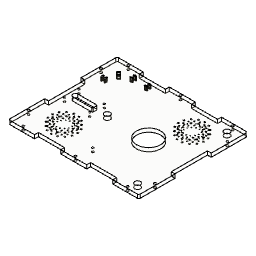
carter_dessous_KOSMOS3-0 (Autodesk Fusion 360 design; units mm, degrees)
Autodesk Fusion 360 part; units mm, degrees
sketch "Esquisse1" plane through (0, 0, 0) normal (0, 0, 1) x (1, 0, 0)
  circle A0 centre (-16.5, 75) radius 16.6
  circle A1 centre (-73.5, 75) radius 3.95
  arc A2 (-133, 150) -> (-135, 148) centre (-133, 148) ccw
  arc A3 (43, 0) -> (45, 2) centre (43, 2) ccw
  arc A4 (45, 148) -> (43, 150) centre (43, 148) ccw
  arc A5 (-135, 2) -> (-133, 0) centre (-133, 2) ccw
  line L0 (-73.5, 75) -> (-16.5, 75) construction
  line L1 (-135, 75) -> (45, 75) construction
  line L2 (-45, 75) -> (40, 145) construction
  circle A6 centre (30, 136.7647) radius 3.95
  circle A7 centre (30, 13.2353) radius 3.95
  line L3 (-63, 0) -> (-63, 5.3)
  line L4 (-63, 5.3) -> (-99, 5.3)
  line L5 (-99, 5.3) -> (-99, 0)
  line L6 (9, 0) -> (9, 5.3)
  line L7 (9, 5.3) -> (-27, 5.3)
  line L8 (-27, 5.3) -> (-27, 0)
  line L9 (-133, 0) -> (-99, 0)
  line L10 (-63, 0) -> (-27, 0)
  line L11 (9, 0) -> (43, 0)
  line L12 (-63, 150) -> (-63, 144.7)
  line L13 (-63, 144.7) -> (-99, 144.7)
  line L14 (-99, 144.7) -> (-99, 150)
  line L15 (9, 150) -> (9, 144.7)
  line L16 (9, 144.7) -> (-27, 144.7)
  line L17 (-27, 144.7) -> (-27, 150)
  line L18 (-133, 150) -> (-99, 150)
  line L19 (-63, 150) -> (-27, 150)
  line L20 (9, 150) -> (43, 150)
  line L21 (-135, 100) -> (-129.7, 100)
  line L22 (-129.7, 100) -> (-129.7, 50)
  line L23 (-129.7, 50) -> (-135, 50)
  line L24 (-135, 100) -> (-135, 148)
  line L25 (-135, 2) -> (-135, 50)
  line L26 (45, 100) -> (39.7, 100)
  line L27 (39.7, 100) -> (39.7, 50)
  line L28 (39.7, 50) -> (45, 50)
  line L29 (45, 148) -> (45, 100)
  line L30 (45, 2) -> (45, 50)
  arc A8 (-117.7, 78.45) -> (-117.7, 71.55) centre (-117.7, 75) ccw
  line L31 (-117.7, 75) -> (-117.7, 78.45) construction
  line L32 (-117.7, 75) -> (-117.7, 71.55) construction
  line L33 (-117.7, 78.45) -> (-91.7, 78.45)
  line L34 (-117.7, 71.55) -> (-91.7, 71.55)
  circle A9 centre (-117, 2.65) radius 1.5
  circle A10 centre (-45, 2.65) radius 1.5
  circle A11 centre (27, 2.65) radius 1.5
  circle A12 centre (-45, 147.35) radius 1.5
  circle A13 centre (-117, 147.35) radius 1.5
  circle A14 centre (27, 147.35) radius 1.5
  circle A15 centre (-132.35, 25) radius 1.5
  circle A16 centre (42.35, 25) radius 1.5
  circle A17 centre (42.35, 125) radius 1.5
  circle A18 centre (-132.35, 125) radius 1.5
  line L35 (-90.7, 77.45) -> (-90.7, 72.55)
  arc A19 (-90.7, 77.45) -> (-91.7, 78.45) centre (-91.7, 77.45) ccw
  arc A20 (-91.7, 71.55) -> (-90.7, 72.55) centre (-91.7, 72.55) ccw
  circle A21 centre (-122.7, 65) radius 1.275
  circle A22 centre (-87.7, 65) radius 1.275
  circle A23 centre (-122.7, 85) radius 1.275
  circle A24 centre (-87.7, 85) radius 1.275
  circle A25 centre (-52.309, 25) radius 15.2 construction
  circle A26 centre (-52.309, 25) radius 9 construction
  circle A27 centre (-43.3157, 24.6541) radius 1.4
  point P0 (-135, 0)
  point P1 (-135, 150)
  point P2 (45, 150)
  point P3 (-90.7, 71.55)
  point P4 (-90.7, 78.45)
  dimension "d1" = 180
  dimension "d2" = 150
  dimension "d5" = 33.2
  dimension "d6" = 7.9
  dimension "d7" = 2
  dimension "d8" = 2
  dimension "d9" = 2
  dimension "d34" = 7.9
  dimension "d41" = 36
  dimension "d42" = 5.3
  dimension "d47" = 36
  dimension "d48" = 36
  dimension "d49" = 5.3
  dimension "d51" = 6.9
  dimension "d52" = 36
  dimension "d53" = 36
  dimension "d55" = 36
  dimension "d56" = 5.3
  dimension "d57" = 5.3
  dimension "d58" = 5.3
  dimension "d59" = 50
  dimension "d60" = 50
  dimension "d61" = 5.3
  dimension "d62" = 50
  dimension "d63" = 50
  dimension "d65" = 180
  dimension "d66" = 12
  dimension "d67" = 3
  dimension "d68" = 2.65
  dimension "d69" = 18
  dimension "d70" = 3
  dimension "d71" = 2.65
  dimension "d72" = 18
  dimension "d73" = 3
  dimension "d74" = 2.65
  dimension "d75" = 18
  dimension "d76" = 3
  dimension "d77" = 25
  dimension "d78" = 2.65
  dimension "d79" = 3
  dimension "d80" = 2.65
  dimension "d81" = 25
  dimension "d118" = 27
  dimension "d119" = 1
  dimension "d120" = 1
  dimension "d121" = 2.55
  dimension "d122" = 2.55
  dimension "d123" = 35
  dimension "d124" = 7
  dimension "d125" = 10
  dimension "d126" = 10
  dimension "d147" = 30.4
  dimension "d148" = 50
  dimension "d149" = 82.691
  dimension "d150" = 18
  dimension "d151" = 2.8
  constraint equal A2 A3
  constraint coincident A1.centre L0.start
  constraint coincident A0.centre L0.end
  constraint midpoint L0 L2.start
  constraint coincident L2 A6.centre
  constraint symmetric L1 A6 A7
  constraint vertical L3
  constraint horizontal L4
  constraint vertical L5
  constraint vertical L6
  constraint horizontal L7
  constraint vertical L8
  constraint tangent A5 L9
  constraint perpendicular L8 L10
  constraint tangent A3 L11
  constraint vertical L12
  constraint horizontal L13
  constraint vertical L14
  constraint vertical L15
  constraint horizontal L16
  constraint vertical L17
  constraint tangent A2 L18
  constraint perpendicular L17 L19
  constraint tangent A4 L20
  constraint horizontal L21
  constraint vertical L22
  constraint horizontal L23
  constraint tangent A2 L24
  constraint tangent A5 L25
  constraint horizontal L26
  constraint vertical L27
  constraint horizontal L28
  constraint tangent A4 L29
  constraint tangent A3 L30
  constraint symmetric L1 A9 A13
  constraint symmetric L1 A10 A12
  constraint symmetric L1 A11 A14
  constraint symmetric L1 A15 A18
  constraint symmetric L1 A16 A17
  constraint perpendicular L34 L35
  constraint coincident P4 L33
  constraint coincident P4 L35
  constraint tangent L33 A19
  constraint tangent L35 A19
  constraint coincident P3 L34
  constraint coincident P3 L35
  constraint tangent L34 A20
  constraint tangent L35 A20
  constraint tangent A8 L34
  constraint parallel L1 L33
  constraint parallel L33 L34
  constraint coincident L1 A8.centre
  constraint symmetric L1 A21 A23
  constraint symmetric L1 A22 A24
  constraint concentric A25 A26
  constraint coincident A26 A27.centre
  measures "d1" distance of P1 P2
  measures "d2" distance of P0 P1
  measures "d5" diameter of A0
  measures "d6" diameter of A1
  measures "d7" radius of A2
  measures "d8" radius of A4
  measures "d9" radius of A5
  measures "d34" diameter of A6
  measures "d41" distance of L3.end L4.end
  measures "d42" distance of L5.end L4.end
  measures "d47" distance of L6.end L7.end
  measures "d48" distance of L3 L8
  measures "d49" distance of L8.end L7.end
  measures "d51" distance of P3 P4
  measures "d52" distance of L12.end L13.end
  measures "d53" distance of L12 L17
  measures "d55" distance of L15.end L16.end
  measures "d56" distance of L14.end L13.end
  measures "d57" distance of L17.end L16.end
  measures "d58" distance of L21.start L21.end
  measures "d59" distance of L21.end L22.end
  measures "d60" distance of L9 L23
  measures "d61" distance of L26.start L26.end
  measures "d62" distance of L26.end L27.end
  measures "d63" distance of L11 L28
  measures "d65" angle of L31 L32
  measures "d66" distance of L22 A8.centre
  measures "d67" diameter of A9
  measures "d68" distance of L9 A9.centre
  measures "d69" distance of L5 A9.centre
  measures "d71" distance of L10 A10.centre
  measures "d72" distance of L3 A10.centre
  measures "d73" diameter of A11
  measures "d74" distance of L11 A11.centre
  measures "d75" distance of L6 A11.centre
  measures "d76" diameter of A15
  measures "d77" distance of L23 A15.centre
  measures "d78" distance of L25 A15.centre
  measures "d79" diameter of A16
  measures "d80" distance of L30 A16.centre
  measures "d81" distance of L28 A16.centre
  measures "d118" distance of P4 A8.start
  measures "d119" radius of A19
  measures "d120" radius of A20
  measures "d121" diameter of A21
  measures "d122" diameter of A22
  measures "d123" distance of A21.centre A22.centre
  measures "d124" distance of L22 A21.centre
  measures "d125" distance of L1 A22.centre
  measures "d126" distance of L1 A21.centre
  measures "d147" diameter of A25
  measures "d148" distance of L1 A25.centre
  measures "d149" distance of L25 A25.centre
  measures "d150" diameter of A26
  measures "d151" diameter of A27
extrude "Extrusion1" add sketch "Esquisse1" along normal blind 5
sketch "Esquisse2" plane through (0, 0, 5) normal (0, 0, 1) x (-1, 0, 0)
  arc A0 (117.7, -78.45) -> (117.7, -71.55) centre (117.7, -75) ccw
  line L0 (117.7, -78.45) -> (91.7, -78.45)
  line L1 (91.7, -71.55) -> (117.7, -71.55)
  circle A1 centre (-42.35, -125) radius 1.5
  circle A2 centre (-42.35, -25) radius 1.5
  circle A3 centre (132.35, -125) radius 1.5
  circle A4 centre (-30, -13.2353) radius 3.95
  circle A5 centre (45, -147.35) radius 1.5
  circle A6 centre (132.35, -25) radius 1.5
  circle A7 centre (-27, -147.35) radius 1.5
  circle A8 centre (117, -147.35) radius 1.5
  circle A9 centre (16.5, -75) radius 16.6
  circle A10 centre (73.5, -75) radius 3.95
  circle A11 centre (-30, -136.7647) radius 3.95
  circle A12 centre (117, -2.65) radius 1.5
  circle A13 centre (45, -2.65) radius 1.5
  circle A14 centre (-27, -2.65) radius 1.5
  line L2 (-9, 0) -> (-43, 0)
  arc A15 (-43, 0) -> (-45, -2) centre (-43, -2) ccw
  line L3 (-45, -2) -> (-45, -50)
  line L4 (-45, -50) -> (-39.7, -50)
  line L5 (-39.7, -50) -> (-39.7, -100)
  line L6 (-39.7, -100) -> (-45, -100)
  line L7 (-45, -100) -> (-45, -148)
  arc A16 (-45, -148) -> (-43, -150) centre (-43, -148) ccw
  line L8 (-43, -150) -> (-9, -150)
  line L9 (-9, -150) -> (-9, -144.7)
  line L10 (-9, -144.7) -> (27, -144.7)
  line L11 (27, -144.7) -> (27, -150)
  line L12 (27, -150) -> (63, -150)
  line L13 (63, -150) -> (63, -144.7)
  line L14 (63, -144.7) -> (99, -144.7)
  line L15 (99, -144.7) -> (99, -150)
  line L16 (99, -150) -> (133, -150)
  arc A17 (133, -150) -> (135, -148) centre (133, -148) ccw
  line L17 (135, -148) -> (135, -100)
  line L18 (135, -100) -> (129.7, -100)
  line L19 (129.7, -100) -> (129.7, -50)
  line L20 (129.7, -50) -> (135, -50)
  line L21 (135, -50) -> (135, -2)
  arc A18 (135, -2) -> (133, 0) centre (133, -2) ccw
  line L22 (133, 0) -> (99, 0)
  line L23 (99, 0) -> (99, -5.3)
  line L24 (99, -5.3) -> (63, -5.3)
  line L25 (63, -5.3) -> (63, 0)
  line L26 (63, 0) -> (27, 0)
  line L27 (27, 0) -> (27, -5.3)
  line L28 (27, -5.3) -> (-9, -5.3)
  line L29 (-9, -5.3) -> (-9, 0)
  circle A19 centre (93.5239, -35) radius 17.5 construction
  circle A20 centre (100.6418, -19.013) radius 1
  circle A21 centre (93.5239, -17.5) radius 1
  circle A22 centre (86.406, -19.013) radius 1
  circle A23 centre (80.5188, -23.2902) radius 1
  circle A24 centre (76.8804, -29.5922) radius 1
  circle A25 centre (76.1197, -36.8292) radius 1
  circle A26 centre (78.3684, -43.75) radius 1
  circle A27 centre (83.2376, -49.1578) radius 1
  circle A28 centre (89.8854, -52.1176) radius 1
  circle A29 centre (97.1623, -52.1176) radius 1
  circle A30 centre (103.8101, -49.1578) radius 1
  circle A31 centre (108.6793, -43.75) radius 1
  circle A32 centre (110.928, -36.8292) radius 1
  circle A33 centre (110.1674, -29.5922) radius 1
  circle A34 centre (106.5289, -23.2902) radius 1
  line L30 (93.5239, -35) -> (93.5239, -5.3) construction
  line L31 (93.5239, -35) -> (100.6418, -19.013) construction
  circle A35 centre (93.5239, -35) radius 14 construction
  line L32 (93.5239, -35) -> (101.7529, -23.6738) construction
  circle A36 centre (101.7529, -23.6738) radius 0.8
  circle A37 centre (96.4346, -21.3059) radius 0.8
  circle A38 centre (90.6131, -21.3059) radius 0.8
  circle A39 centre (85.2949, -23.6738) radius 0.8
  circle A40 centre (81.3995, -28) radius 0.8
  circle A41 centre (79.6006, -33.5366) radius 0.8
  circle A42 centre (80.2091, -39.3262) radius 0.8
  circle A43 centre (83.1199, -44.3678) radius 0.8
  circle A44 centre (87.8296, -47.7896) radius 0.8
  circle A45 centre (93.5239, -49) radius 0.8
  circle A46 centre (99.2182, -47.7896) radius 0.8
  circle A47 centre (103.9279, -44.3678) radius 0.8
  circle A48 centre (106.8387, -39.3262) radius 0.8
  circle A49 centre (107.4472, -33.5366) radius 0.8
  circle A50 centre (105.6482, -28) radius 0.8
  circle A51 centre (93.5239, -35) radius 10.5 construction
  circle A52 centre (97.7946, -25.4078) radius 0.6
  circle A53 centre (93.5239, -24.5) radius 0.6
  circle A54 centre (89.2531, -25.4078) radius 0.6
  circle A55 centre (85.7209, -27.9741) radius 0.6
  circle A56 centre (83.5378, -31.7553) radius 0.6
  circle A57 centre (83.0814, -36.0975) radius 0.6
  circle A58 centre (84.4306, -40.25) radius 0.6
  circle A59 centre (87.3521, -43.4947) radius 0.6
  circle A60 centre (91.3408, -45.2705) radius 0.6
  circle A61 centre (95.707, -45.2705) radius 0.6
  circle A62 centre (99.6956, -43.4947) radius 0.6
  circle A63 centre (102.6171, -40.25) radius 0.6
  circle A64 centre (103.9664, -36.0975) radius 0.6
  circle A65 centre (103.51, -31.7553) radius 0.6
  circle A66 centre (101.3269, -27.9741) radius 0.6
  line L33 (156.7045, -75) -> (-43.2955, -75) construction
  line L34 (45, -161.7716) -> (45, 30) construction
  line L35 (-76.1475, -174.8663) -> (45, -75) construction
  line L36 (-76.1475, -174.8663) -> (225.7956, 74.0364) construction
  circle A67 centre (-7.7946, -124.5922) radius 0.6
  circle A68 centre (-3.5239, -115) radius 10.5 construction
  circle A69 centre (8.6005, -122) radius 0.8
  circle A70 centre (-18.6793, -106.25) radius 1
  circle A71 centre (-13.9279, -105.6322) radius 0.8
  circle A72 centre (4.7051, -126.3262) radius 0.8
  circle A73 centre (-16.8387, -110.6738) radius 0.8
  circle A74 centre (-15.6482, -122) radius 0.8
  circle A75 centre (-13.8101, -100.8422) radius 1
  circle A76 centre (-9.2182, -102.2104) radius 0.8
  circle A77 centre (-3.5239, -101) radius 0.8
  circle A78 centre (-13.51, -118.2447) radius 0.6
  circle A79 centre (-9.6956, -106.5053) radius 0.6
  circle A80 centre (-10.6418, -130.987) radius 1
  circle A81 centre (-1.3408, -104.7295) radius 0.6
  circle A82 centre (-16.5289, -126.7098) radius 1
  circle A83 centre (0.7469, -124.5922) radius 0.6
  circle A84 centre (10.3994, -116.4634) radius 0.8
  circle A85 centre (13.1196, -120.4078) radius 1
  circle A86 centre (13.8803, -113.1708) radius 1
  circle A87 centre (11.6316, -106.25) radius 1
  circle A88 centre (6.8801, -105.6322) radius 0.8
  circle A89 centre (3.594, -130.987) radius 1
  circle A90 centre (-20.1674, -120.4078) radius 1
  circle A91 centre (-5.707, -104.7295) radius 0.6
  circle A92 centre (-3.5239, -125.5) radius 0.6
  circle A93 centre (-0.6131, -128.6941) radius 0.8
  circle A94 centre (-3.5239, -132.5) radius 1
  circle A95 centre (-12.6171, -109.75) radius 0.6
  circle A96 centre (4.2791, -122.0259) radius 0.6
  circle A97 centre (6.9186, -113.9025) radius 0.6
  circle A98 centre (-11.7529, -126.3262) radius 0.8
  circle A99 centre (-6.4346, -128.6941) radius 0.8
  circle A100 centre (-20.928, -113.1708) radius 1
  circle A101 centre (6.7624, -100.8422) radius 1
  circle A102 centre (0.1146, -97.8824) radius 1
  circle A103 centre (2.1704, -102.2104) radius 0.8
  circle A104 centre (2.6479, -106.5053) radius 0.6
  line L37 (-3.5239, -115) -> (-10.6418, -130.987) construction
  line L38 (-3.5239, -115) -> (-11.7529, -126.3262) construction
  circle A105 centre (6.4622, -118.2447) radius 0.6
  circle A106 centre (5.5694, -109.75) radius 0.6
  circle A107 centre (-7.1623, -97.8824) radius 1
  circle A108 centre (-13.9664, -113.9025) radius 0.6
  circle A109 centre (9.4812, -126.7098) radius 1
  circle A110 centre (-11.3269, -122.0259) radius 0.6
  circle A111 centre (-3.5239, -115) radius 14 construction
  circle A112 centre (-3.5239, -115) radius 17.5 construction
  circle A113 centre (-17.4472, -116.4634) radius 0.8
  circle A114 centre (9.7909, -110.6738) radius 0.8
  arc A115 (90.7, -77.45) -> (91.7, -78.45) centre (91.7, -77.45) ccw
  line L39 (90.7, -77.45) -> (90.7, -72.55)
  arc A116 (91.7, -71.55) -> (90.7, -72.55) centre (91.7, -72.55) ccw
  circle A117 centre (122.7, -85) radius 1.275
  circle A118 centre (87.7, -85) radius 1.275
  circle A119 centre (87.7, -65) radius 1.275
  circle A120 centre (122.7, -65) radius 1.275
  circle A121 centre (43.3157, -24.6541) radius 1.4
  dimension "d83" = 35
  dimension "d84" = 2
  dimension "d87" = 24
  dimension "d88" = 28
  dimension "d90" = 1.6
  dimension "d93" = 21
  dimension "d95" = 1.2
  dimension "d111" = 40
  dimension "d114" = 39.5
  constraint coincident A19 A20.centre
  constraint coincident A19.centre L30.start
  constraint coincident L24 L30.end
  constraint perpendicular L24 L30
  constraint coincident A20.centre L31.end
  constraint coincident A35 L32.end
  constraint coincident L32.end A36.centre
  constraint coincident A51 A52.centre
  constraint coincident L31 A52.centre
  constraint perpendicular L5 L33
  constraint perpendicular L24 L34
  constraint coincident L33 L35.end
  constraint coincident L34 L35.end
  constraint parallel L35 L36
  constraint coincident A19.centre L36
  measures "d83" diameter of A19
  measures "d84" diameter of A20
  measures "d87" angle of L30 L31
  measures "d88" diameter of A35
  measures "d90" diameter of A36
  measures "d93" diameter of A51
  measures "d95" diameter of A52
  measures "d111" distance of A19.centre L33
  measures "d114" angle of L33 L35
extrude "Extrusion2" cut sketch "Esquisse2" against normal blind 5 contours A20 | A21 | A22 | A23 | A24 | A25 | A26 | A27 | A28 | A29 | A30 | A31 | A32 | A33 | A34 | A36 | A37 | A38 | A39 | A40 | A41 | A42 | A43 | A44 | A45 | A46 | A47 | A48 | A49 | A50 | A52 | A53 | A54 | A55 | A56 | A57 | A58 | A59 | A60 | A61 | A62 | A63 | A64 | A65 | A66 | A67 | A69 | A70 | A71 | A72 | A73 | A74 | A75 | A76 | A77 | A78 | A79 | A80 | A81 | A82 | A83 | A84 | A85 | A86 | A87 | A88 | A89 | A90 | A91 | A92 | A93 | A94 | A95 | A96 | A97 | A98 | A99 | A100 | A101 | A102 | A103 | A104 | A105 | A106 | A107 | A108 | A109 | A110 | A113 | A114
sketch "Esquisse3" plane through (0, 0, 5) normal (0, 0, 1) x (-1, 0, 0)
  circle A0 centre (-1.3408, -104.7295) radius 0.6
  circle A1 centre (4.7051, -126.3262) radius 0.8
  circle A2 centre (6.8801, -105.6322) radius 0.8
  circle A3 centre (6.9186, -113.9025) radius 0.6
  circle A4 centre (-9.2182, -102.2104) radius 0.8
  circle A5 centre (-6.4346, -128.6941) radius 0.8
  circle A6 centre (0.7469, -124.5922) radius 0.6
  circle A7 centre (0.1146, -97.8824) radius 1
  circle A8 centre (-20.928, -113.1708) radius 1
  circle A9 centre (-0.6131, -128.6941) radius 0.8
  circle A10 centre (5.5694, -109.75) radius 0.6
  circle A11 centre (89.8854, -52.1176) radius 1
  circle A12 centre (85.2949, -23.6738) radius 0.8
  circle A13 centre (86.406, -19.013) radius 1
  circle A14 centre (85.7209, -27.9741) radius 0.6
  circle A15 centre (103.8101, -49.1578) radius 1
  circle A16 centre (103.9279, -44.3678) radius 0.8
  circle A17 centre (106.8387, -39.3262) radius 0.8
  circle A18 centre (103.9664, -36.0975) radius 0.6
  circle A19 centre (95.707, -45.2705) radius 0.6
  circle A20 centre (99.6956, -43.4947) radius 0.6
  circle A21 centre (83.1199, -44.3678) radius 0.8
  circle A22 centre (79.6006, -33.5366) radius 0.8
  circle A23 centre (87.8296, -47.7896) radius 0.8
  circle A24 centre (110.1674, -29.5922) radius 1
  circle A25 centre (108.6793, -43.75) radius 1
  circle A26 centre (91.3408, -45.2705) radius 0.6
  circle A27 centre (106.5289, -23.2902) radius 1
  circle A28 centre (93.5239, -49) radius 0.8
  circle A29 centre (101.3269, -27.9741) radius 0.6
  circle A30 centre (83.2376, -49.1578) radius 1
  circle A31 centre (96.4346, -21.3059) radius 0.8
  circle A32 centre (76.8804, -29.5922) radius 1
  circle A33 centre (76.1197, -36.8292) radius 1
  circle A34 centre (2.1704, -102.2104) radius 0.8
  circle A35 centre (2.6479, -106.5053) radius 0.6
  circle A36 centre (-3.5239, -101) radius 0.8
  circle A37 centre (11.6316, -106.25) radius 1
  circle A38 centre (9.7909, -110.6738) radius 0.8
  circle A39 centre (-15.6482, -122) radius 0.8
  circle A40 centre (-18.6793, -106.25) radius 1
  circle A41 centre (-16.5289, -126.7098) radius 1
  circle A42 centre (3.594, -130.987) radius 1
  circle A43 centre (10.3994, -116.4634) radius 0.8
  circle A44 centre (8.6005, -122) radius 0.8
  circle A45 centre (-7.7946, -124.5922) radius 0.6
  circle A46 centre (13.8803, -113.1708) radius 1
  circle A47 centre (6.7624, -100.8422) radius 1
  circle A48 centre (-13.9279, -105.6322) radius 0.8
  circle A49 centre (-13.51, -118.2447) radius 0.6
  circle A50 centre (4.2791, -122.0259) radius 0.6
  circle A51 centre (-20.1674, -120.4078) radius 1
  circle A52 centre (-17.4472, -116.4634) radius 0.8
  circle A53 centre (-13.9664, -113.9025) radius 0.6
  circle A54 centre (-10.6418, -130.987) radius 1
  circle A55 centre (6.4622, -118.2447) radius 0.6
  circle A56 centre (81.3995, -28) radius 0.8
  circle A57 centre (97.1623, -52.1176) radius 1
  circle A58 centre (80.5188, -23.2902) radius 1
  circle A59 centre (89.2531, -25.4078) radius 0.6
  circle A60 centre (83.5378, -31.7553) radius 0.6
  circle A61 centre (107.4472, -33.5366) radius 0.8
  circle A62 centre (105.6482, -28) radius 0.8
  circle A63 centre (110.928, -36.8292) radius 1
  circle A64 centre (84.4306, -40.25) radius 0.6
  circle A65 centre (100.6418, -19.013) radius 1
  circle A66 centre (80.2091, -39.3262) radius 0.8
  circle A67 centre (101.7529, -23.6738) radius 0.8
  circle A68 centre (78.3684, -43.75) radius 1
  circle A69 centre (102.6171, -40.25) radius 0.6
  circle A70 centre (87.3521, -43.4947) radius 0.6
  circle A71 centre (103.51, -31.7553) radius 0.6
  circle A72 centre (83.0814, -36.0975) radius 0.6
  circle A73 centre (99.2182, -47.7896) radius 0.8
  circle A74 centre (93.5239, -24.5) radius 0.6
  circle A75 centre (93.5239, -17.5) radius 1
  circle A76 centre (97.7946, -25.4078) radius 0.6
  circle A77 centre (90.6131, -21.3059) radius 0.8
  circle A78 centre (-9.6956, -106.5053) radius 0.6
  circle A79 centre (-3.5239, -132.5) radius 1
  circle A80 centre (-7.1623, -97.8824) radius 1
  circle A81 centre (-11.3269, -122.0259) radius 0.6
  circle A82 centre (13.1196, -120.4078) radius 1
  circle A83 centre (-13.8101, -100.8422) radius 1
  circle A84 centre (9.4812, -126.7098) radius 1
  circle A85 centre (-16.8387, -110.6738) radius 0.8
  circle A86 centre (-3.5239, -125.5) radius 0.6
  circle A87 centre (-5.707, -104.7295) radius 0.6
  circle A88 centre (-12.6171, -109.75) radius 0.6
  circle A89 centre (-11.7529, -126.3262) radius 0.8
  arc A90 (117.7, -78.45) -> (117.7, -71.55) centre (117.7, -75) ccw
  line L0 (117.7, -78.45) -> (91.7, -78.45)
  arc A91 (90.7, -77.45) -> (91.7, -78.45) centre (91.7, -77.45) ccw
  line L1 (90.7, -77.45) -> (90.7, -72.55)
  arc A92 (91.7, -71.55) -> (90.7, -72.55) centre (91.7, -72.55) ccw
  line L2 (91.7, -71.55) -> (117.7, -71.55)
  circle A93 centre (122.7, -65) radius 1.275
  circle A94 centre (132.35, -125) radius 1.5
  circle A95 centre (87.7, -65) radius 1.275
  circle A96 centre (-27, -147.35) radius 1.5
  circle A97 centre (-42.35, -125) radius 1.5
  circle A98 centre (-30, -13.2353) radius 3.95
  circle A99 centre (117, -2.65) radius 1.5
  circle A100 centre (45, -2.65) radius 1.5
  circle A101 centre (132.35, -25) radius 1.5
  circle A102 centre (16.5, -75) radius 16.6
  circle A103 centre (-30, -136.7647) radius 3.95
  circle A104 centre (122.7, -85) radius 1.275
  circle A105 centre (-27, -2.65) radius 1.5
  circle A106 centre (45, -147.35) radius 1.5
  circle A107 centre (87.7, -85) radius 1.275
  circle A108 centre (117, -147.35) radius 1.5
  circle A109 centre (73.5, -75) radius 3.95
  circle A110 centre (-42.35, -25) radius 1.5
  line L3 (-9, 0) -> (-43, 0)
  arc A111 (-43, 0) -> (-45, -2) centre (-43, -2) ccw
  line L4 (-45, -2) -> (-45, -50)
  line L5 (-45, -50) -> (-39.7, -50)
  line L6 (-39.7, -50) -> (-39.7, -100)
  line L7 (-39.7, -100) -> (-45, -100)
  line L8 (-45, -100) -> (-45, -148)
  arc A112 (-45, -148) -> (-43, -150) centre (-43, -148) ccw
  line L9 (-43, -150) -> (-9, -150)
  line L10 (-9, -150) -> (-9, -144.7)
  line L11 (-9, -144.7) -> (27, -144.7)
  line L12 (27, -144.7) -> (27, -150)
  line L13 (27, -150) -> (63, -150)
  line L14 (63, -150) -> (63, -144.7)
  line L15 (63, -144.7) -> (99, -144.7)
  line L16 (99, -144.7) -> (99, -150)
  line L17 (99, -150) -> (133, -150)
  arc A113 (133, -150) -> (135, -148) centre (133, -148) ccw
  line L18 (135, -148) -> (135, -100)
  line L19 (135, -100) -> (129.7, -100)
  line L20 (129.7, -100) -> (129.7, -50)
  line L21 (129.7, -50) -> (135, -50)
  line L22 (135, -50) -> (135, -2)
  arc A114 (135, -2) -> (133, 0) centre (133, -2) ccw
  line L23 (133, 0) -> (99, 0)
  line L24 (99, 0) -> (99, -5.3)
  line L25 (99, -5.3) -> (63, -5.3)
  line L26 (63, -5.3) -> (63, 0)
  line L27 (63, 0) -> (27, 0)
  line L28 (27, 0) -> (27, -5.3)
  line L29 (27, -5.3) -> (-9, -5.3)
  line L30 (-9, -5.3) -> (-9, 0)
  line L31 (117.5, -119) -> (123, -119)
  line L32 (123, -119) -> (123, -115)
  line L33 (122.5, -115) -> (117.5, -115)
  line L34 (117, -115) -> (117, -118.5)
  line L35 (123, -115) -> (122, -115)
  line L36 (121.5, -115.5) -> (121.5, -118.5)
  line L37 (122, -119) -> (122.5, -119)
  line L38 (123, -118.5) -> (123, -115.5)
  line L39 (117, -115) -> (118, -115)
  line L40 (118.5, -115.5) -> (118.5, -118.5)
  line L41 (118, -119) -> (117, -119)
  line L42 (117, -119) -> (117, -115.5)
  arc A115 (122.5, -119) -> (123, -118.5) centre (122.5, -118.5) ccw
  arc A116 (121.5, -118.5) -> (122, -119) centre (122, -118.5) ccw
  arc A117 (122, -115) -> (121.5, -115.5) centre (122, -115.5) ccw
  arc A118 (123, -115.5) -> (122.5, -115) centre (122.5, -115.5) ccw
  arc A119 (118.5, -115.5) -> (118, -115) centre (118, -115.5) ccw
  arc A120 (117.5, -115) -> (117, -115.5) centre (117.5, -115.5) ccw
  arc A121 (117, -118.5) -> (117.5, -119) centre (117.5, -118.5) ccw
  arc A122 (118, -119) -> (118.5, -118.5) centre (118, -118.5) ccw
  arc A123 (99.8904, -137.1266) -> (119.5169, -117.5) centre (99.8904, -117.5) ccw construction
  line L43 (99.8904, -117.5) -> (99.8904, -137.1266) construction
  line L44 (99.8904, -117.5) -> (119.5169, -117.5) construction
  line L45 (98.3904, -135.6096) -> (98.3904, -134.6096)
  line L46 (102.3904, -140.1096) -> (102.3904, -135.1096)
  line L47 (98.8904, -140.6096) -> (101.8904, -140.6096)
  arc A124 (98.8904, -139.1096) -> (98.3904, -139.6096) centre (98.8904, -139.6096) ccw
  line L48 (98.3904, -134.6096) -> (101.8904, -134.6096)
  line L49 (102.3904, -134.6096) -> (102.3904, -135.6096)
  line L50 (98.3904, -140.6096) -> (102.3904, -140.6096)
  line L51 (101.8904, -136.1096) -> (98.8904, -136.1096)
  arc A125 (98.8904, -134.6096) -> (98.3904, -135.1096) centre (98.8904, -135.1096) ccw
  arc A126 (101.8904, -136.1096) -> (102.3904, -135.6096) centre (101.8904, -135.6096) ccw
  arc A127 (102.3904, -139.6096) -> (101.8904, -139.1096) centre (101.8904, -139.6096) ccw
  line L52 (101.8904, -139.1096) -> (98.8904, -139.1096)
  line L53 (102.3904, -134.6096) -> (98.8904, -134.6096)
  line L54 (102.3904, -140.6096) -> (102.3904, -139.6096)
  line L55 (98.3904, -135.1096) -> (98.3904, -140.6096)
  arc A128 (101.8904, -140.6096) -> (102.3904, -140.1096) centre (101.8904, -140.1096) ccw
  arc A129 (102.3904, -135.1096) -> (101.8904, -134.6096) centre (101.8904, -135.1096) ccw
  arc A130 (98.3904, -135.6096) -> (98.8904, -136.1096) centre (98.8904, -135.6096) ccw
  arc A131 (98.3904, -140.1096) -> (98.8904, -140.6096) centre (98.8904, -140.1096) ccw
  line L56 (98.3904, -139.6096) -> (98.3904, -140.1096)
  line L57 (115.1707, -134.9016) -> (117.9991, -132.0732)
  arc A132 (117.292, -131.3661) -> (116.5849, -131.3661) centre (116.9384, -131.7197) ccw
  line L58 (117.6456, -131.7197) -> (114.11, -128.1841)
  line L59 (110.928, -130.659) -> (113.4029, -128.1841)
  arc A133 (114.8171, -134.5481) -> (115.5242, -134.5481) centre (115.1707, -134.1945) ccw
  line L60 (116.5849, -131.3661) -> (114.4636, -133.4874)
  line L61 (113.7565, -127.8306) -> (114.4636, -128.5377)
  arc A134 (111.2816, -130.3055) -> (111.2816, -131.0126) centre (111.6351, -130.659) ccw
  line L62 (113.7565, -127.8306) -> (111.2816, -130.3055)
  arc A135 (114.4636, -129.2448) -> (114.4636, -128.5377) centre (114.11, -128.8912) ccw
  line L63 (111.2816, -131.0126) -> (115.1707, -134.9016)
  line L64 (114.4636, -129.2448) -> (112.3423, -131.3661)
  line L65 (114.4636, -134.1945) -> (114.8171, -134.5481)
  arc A136 (117.6456, -132.4268) -> (117.6456, -131.7197) centre (117.292, -132.0732) ccw
  arc A137 (111.6351, -131.3661) -> (112.3423, -131.3661) centre (111.9887, -131.0126) ccw
  line L66 (115.5242, -134.5481) -> (117.6456, -132.4268)
  arc A138 (114.4636, -133.4874) -> (114.4636, -134.1945) centre (114.8171, -133.841) ccw
  line L67 (111.6351, -131.3661) -> (110.928, -130.659)
  arc A139 (114.11, -128.1841) -> (113.4029, -128.1841) centre (113.7565, -128.5377) ccw
  line L68 (117.9991, -132.0732) -> (117.292, -131.3661)
  line L69 (98.3904, -140.6096) -> (102.3904, -140.6096)
  arc A140 (102.3904, -139.6096) -> (101.8904, -139.1096) centre (101.8904, -139.6096) ccw
  line L70 (102.3904, -140.1096) -> (102.3904, -135.1096)
  line L71 (98.3904, -134.6096) -> (101.8904, -134.6096)
  arc A141 (98.3904, -140.1096) -> (98.8904, -140.6096) centre (98.8904, -140.1096) ccw
  line L72 (101.8904, -139.1096) -> (98.8904, -139.1096)
  line L73 (102.3904, -134.6096) -> (102.3904, -135.6096)
  arc A142 (98.8904, -134.6096) -> (98.3904, -135.1096) centre (98.8904, -135.1096) ccw
  line L74 (102.3904, -134.6096) -> (98.8904, -134.6096)
  arc A143 (101.8904, -136.1096) -> (102.3904, -135.6096) centre (101.8904, -135.6096) ccw
  line L75 (98.3904, -135.1096) -> (98.3904, -140.6096)
  line L76 (101.8904, -136.1096) -> (98.8904, -136.1096)
  line L77 (98.3904, -139.6096) -> (98.3904, -140.1096)
  arc A144 (101.8904, -140.6096) -> (102.3904, -140.1096) centre (101.8904, -140.1096) ccw
  arc A145 (98.3904, -135.6096) -> (98.8904, -136.1096) centre (98.8904, -135.6096) ccw
  line L78 (98.8904, -140.6096) -> (101.8904, -140.6096)
  arc A146 (98.8904, -139.1096) -> (98.3904, -139.6096) centre (98.8904, -139.6096) ccw
  line L79 (98.3904, -135.6096) -> (98.3904, -134.6096)
  arc A147 (102.3904, -135.1096) -> (101.8904, -134.6096) centre (101.8904, -135.1096) ccw
  line L80 (102.3904, -140.6096) -> (102.3904, -139.6096)
  line L81 (77, -150) -> (77, -105) construction
  arc A148 (78.8904, -134.6096) -> (78.3904, -135.1096) centre (78.8904, -135.1096) ccw
  line L82 (82.3904, -134.6096) -> (82.3904, -135.6096)
  line L83 (78.3904, -139.6096) -> (78.3904, -140.1096)
  line L84 (82.3904, -140.6096) -> (82.3904, -139.6096)
  line L85 (81.8904, -139.1096) -> (78.8904, -139.1096)
  arc A149 (81.8904, -140.6096) -> (82.3904, -140.1096) centre (81.8904, -140.1096) ccw
  line L86 (78.8904, -140.6096) -> (81.8904, -140.6096)
  arc A150 (82.3904, -139.6096) -> (81.8904, -139.1096) centre (81.8904, -139.6096) ccw
  line L87 (78.8904, -140.6096) -> (81.8904, -140.6096)
  arc A151 (78.8904, -139.1096) -> (78.3904, -139.6096) centre (78.8904, -139.6096) ccw
  arc A152 (82.3904, -135.1096) -> (81.8904, -134.6096) centre (81.8904, -135.1096) ccw
  arc A153 (78.8904, -139.1096) -> (78.3904, -139.6096) centre (78.8904, -139.6096) ccw
  arc A154 (78.8904, -134.6096) -> (78.3904, -135.1096) centre (78.8904, -135.1096) ccw
  arc A155 (82.3904, -139.6096) -> (81.8904, -139.1096) centre (81.8904, -139.6096) ccw
  arc A156 (78.3904, -140.1096) -> (78.8904, -140.6096) centre (78.8904, -140.1096) ccw
  line L88 (82.3904, -140.6096) -> (82.3904, -139.6096)
  arc A157 (81.8904, -140.6096) -> (82.3904, -140.1096) centre (81.8904, -140.1096) ccw
  line L89 (78.3904, -140.6096) -> (82.3904, -140.6096)
  line L90 (82.3904, -134.6096) -> (82.3904, -135.6096)
  arc A158 (78.3904, -140.1096) -> (78.8904, -140.6096) centre (78.8904, -140.1096) ccw
  line L91 (81.8904, -139.1096) -> (78.8904, -139.1096)
  line L92 (78.3904, -139.6096) -> (78.3904, -140.1096)
  line L93 (78.3904, -134.6096) -> (81.8904, -134.6096)
  line L94 (78.3904, -135.6096) -> (78.3904, -134.6096)
  arc A159 (78.3904, -135.6096) -> (78.8904, -136.1096) centre (78.8904, -135.6096) ccw
  arc A160 (82.3904, -135.1096) -> (81.8904, -134.6096) centre (81.8904, -135.1096) ccw
  line L95 (82.3904, -134.6096) -> (78.8904, -134.6096)
  line L96 (82.3904, -140.1096) -> (82.3904, -135.1096)
  line L97 (78.3904, -134.6096) -> (81.8904, -134.6096)
  line L98 (78.3904, -140.6096) -> (82.3904, -140.6096)
  line L99 (78.3904, -135.6096) -> (78.3904, -134.6096)
  arc A161 (81.8904, -136.1096) -> (82.3904, -135.6096) centre (81.8904, -135.6096) ccw
  line L100 (78.3904, -135.1096) -> (78.3904, -140.6096)
  arc A162 (81.8904, -136.1096) -> (82.3904, -135.6096) centre (81.8904, -135.6096) ccw
  line L101 (81.8904, -136.1096) -> (78.8904, -136.1096)
  line L102 (82.3904, -134.6096) -> (78.8904, -134.6096)
  line L103 (81.8904, -136.1096) -> (78.8904, -136.1096)
  arc A163 (78.3904, -135.6096) -> (78.8904, -136.1096) centre (78.8904, -135.6096) ccw
  line L104 (78.3904, -135.1096) -> (78.3904, -140.6096)
  line L105 (82.3904, -140.1096) -> (82.3904, -135.1096)
  circle A164 centre (43.3157, -24.6541) radius 1.4
  point P0 (117, -119)
  point P1 (121.5, -115)
  point P2 (118.5, -115)
  point P3 (102.3904, -139.1096)
  point P4 (102.3904, -136.1096)
  point P5 (99.8904, -137.1266)
  point P6 (98.3904, -134.6096)
  point P7 (116.9384, -131.0126)
  point P8 (113.7684, -131.3781)
  point P9 (110.928, -130.659)
  point P10 (114.8171, -128.8912)
  point P11 (102.3904, -139.1096)
  point P12 (99.8904, -137.1266)
  point P13 (98.3904, -134.6096)
  point P14 (102.3904, -136.1096)
  point P15 (82.3904, -139.1096)
  point P16 (79.8904, -137.1266)
  point P17 (82.3904, -139.1096)
  point P18 (82.3904, -136.1096)
  point P19 (82.3904, -136.1096)
  point P20 (78.3904, -134.6096)
  point P21 (79.8904, -137.1266)
  point P22 (79.8904, -137.1266)
  point P23 (78.3904, -134.6096)
  dimension "d127" = 6
  dimension "d128" = 4
  dimension "d129" = 12
  dimension "d130" = 1.5
  dimension "d131" = 1.5
  dimension "d134" = 0.5
  dimension "d135" = 90
  dimension "d136" = 1.5
  dimension "d138" = 90
  dimension "d139" = 15
  dimension "d141" = -90
  dimension "d142" = 58
  dimension "d145" = -20
  dimension "d146" = 0
  constraint horizontal L31
  constraint vertical L32
  constraint horizontal L33
  constraint vertical L34
  constraint horizontal L35
  constraint vertical L36
  constraint horizontal L37
  constraint vertical L38
  constraint horizontal L39
  constraint vertical L40
  constraint horizontal L41
  constraint vertical L42
  constraint tangent L37 A115
  constraint tangent L38 A115
  constraint tangent L36 A116
  constraint tangent L37 A116
  constraint equal A115 A116
  constraint coincident P1 L35
  constraint coincident P1 L36
  constraint tangent L35 A117
  constraint tangent L36 A117
  constraint equal A115 A117
  constraint coincident L32.end L33
  constraint coincident L32.end L38
  constraint tangent L33 A118
  constraint tangent L38 A118
  constraint equal A115 A118
  constraint coincident P2 L39
  constraint coincident P2 L40
  constraint tangent L39 A119
  constraint tangent L40 A119
  constraint equal A115 A119
  constraint coincident L34.start L33
  constraint coincident L34.start L42
  constraint tangent L33 A120
  constraint tangent L42 A120
  constraint equal A115 A120
  constraint coincident P0 L34
  constraint coincident P0 L31
  constraint tangent L34 A121
  constraint tangent L31 A121
  constraint equal A115 A121
  constraint tangent L40 A122
  constraint tangent L41 A122
  constraint equal A115 A122
  constraint parallel L31 L44
  constraint coincident L41 L31.start
  constraint coincident L31.end L37
  constraint perpendicular L15 L81
  measures "d127" distance of P0 L31.end
  measures "d128" distance of P0 L34.start
  measures "d129" distance of L18 L32
  measures "d130" distance of L32.end P1
  measures "d131" distance of L34.start P2
  measures "d135" angle of L43 L44
  measures "d136" distance of L31 L44
  measures "d139" distance of L19 L33
  measures "d142" distance of L18 L81
extrude "Extrusion3" cut sketch "Esquisse3" against normal blind 5 contours L31 L33 L34 L39 L40 L41 L42 A119 A120 A121 A122 | L31 L32 L33 L35 L36 L37 L38 A115 A116 A117 A118 | L45 L46 L48 L49 L51 A125 A126 L53 L55 A129 A130 L70 L71 L73 A142 L74 A143 L75 L76 A145 L79 A147 | L46 L47 A124 L50 A127 L52 L54 L55 A128 A131 L56 L69 A140 L70 A141 L72 L75 L77 A144 L78 A146 L80 | L57 A132 L58 A133 L60 L63 L65 A136 L66 A138 L68 | L58 L59 L61 A134 L62 A135 L63 L64 A137 L67 A139 | A148 L82 A152 A154 L90 L93 L94 A159 A160 L95 L96 L97 L99 A161 L100 A162 L101 L102 L103 A163 L104 L105 | L83 L84 L85 A149 L86 A150 L87 A151 A153 A155 A156 L88 A157 L89 A158 L91 L92 L96 L98 L100 L104 L105
equation "d47 = d41"
equation "d48 = d41"
equation "d49 = d42"
equation "d52 = d41"
equation "d53 = d52"
equation "d56 = d42"
equation "d57 = d56"
equation "d58 = d42"
equation "d60 = d59"
equation "d62 = d59"
equation "d63 = d62"
equation "d68 = d42 / 2"
equation "d69 = d41 / 2"
equation "d71 = d42 / 2"
equation "d72 = d41 / 2"
equation "d74 = d42 / 2"
equation "d75 = d41 / 2"
equation "d77 = d59 / 2"
equation "d78 = d42 / 2"
equation "d80 = d61 / 2"
equation "d81 = d63 / 2"
equation "d90 = d84 - 0.4 mm"
equation "d95 = d84 - 0.8 mm"
equation "d119 = d120"
equation "d122 = d121"
equation "d126 = d125"
